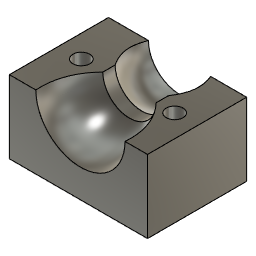
Arm0_1 (Autodesk Fusion 360 design; units mm, degrees)
Autodesk Fusion 360 part; units mm, degrees
note: some values were not read from the file. Set by a fixed rule: which sketch regions a step uses.
sketch "Sketch1" plane through (0, 0, 0) normal (0, 0, 1) x (1, 0, 0)
  line L0 (0.0319, -0.0588) -> (7.7319, -0.0588)
  line L1 (0.0319, 17.6912) -> (0.0319, -0.0588)
  line L2 (0.0319, 17.6912) -> (5.3319, 17.6912)
  line L3 (0.0319, 8.7412) -> (4.5319, 8.7412)
  line L4 (4.5319, 10.9412) -> (0.0319, 10.9412)
  spline S0 degree 5 poles (5.3319, 17.6912) (5.3878, 17.5532) (5.4935, 17.2775) (5.633, 16.8647) (5.7805, 16.3159) (5.8962, 15.6328) (5.9374, 14.9527) (5.8981, 14.2761) (5.7753, 13.6028) (5.5729, 12.9329) (5.297, 12.2661) (5.0223, 11.7348) (4.7879, 11.3376) (4.6193, 11.0732) (4.5319, 10.9412) knots 0 0 0 0 0 0 0.1 0.2 0.3 0.4 0.5 0.6 0.7 0.8 0.9 1 1 1 1 1 1
  line L5 (0.0319, 10.9412) -> (4.5319, 10.9412)
  arc A0 (7.7319, -0.0588) -> (4.5319, 8.7412) centre (-3.0926, 0.9869) ccw
  line L6 (4.5319, 8.7412) -> (4.5319, 10.9412)
  line L7 (0.0319, 10.9412) -> (0.0319, 8.7412)
  line L8 (0.0319, 10.9412) -> (0.0319, 8.7412)
  line L9 (0.0319, 14.3162) -> (5.8819, 14.3162)
  line L10 (0.0319, 17.6912) -> (0.0319, 10.9412)
  line L11 (7.7319, -0.0588) -> (7.9819, -0.0588)
  line L12 (4.5319, 8.7412) -> (4.7819, 8.7412)
  line L13 (4.5319, 10.9412) -> (4.7819, 10.9412)
  line L14 (5.8819, 14.3162) -> (6.1319, 14.3162)
  line L15 (5.3319, 17.6912) -> (5.5819, 17.6912)
  spline S1 degree 5 poles (5.5819, 17.6912) (5.6378, 17.5532) (5.7435, 17.2775) (5.883, 16.8647) (6.0305, 16.3159) (6.1462, 15.6328) (6.1874, 14.9527) (6.1481, 14.2761) (6.0253, 13.6028) (5.8229, 12.9329) (5.547, 12.2661) (5.2723, 11.7348) (5.0379, 11.3376) (4.8693, 11.0732) (4.7819, 10.9412) knots 0 0 0 0 0 0 0.1 0.2 0.3 0.4 0.5 0.6 0.7 0.8 0.9 1 1 1 1 1 1
  line L16 (4.7819, 10.9412) -> (4.7819, 8.7412)
  arc A1 (7.9819, -0.0588) -> (4.7819, 8.7412) centre (-2.9749, 0.9388) ccw
  line L17 (5.5819, 17.6912) -> (9, 17.6912)
  line L18 (9, 17.6912) -> (12, 17.6912)
  line L19 (12, 17.6912) -> (12, 0)
  line L20 (12, 0) -> (7.9819, -0.0588)
  dimension "d1" = 5.3
  dimension "d2" = 6.75
  dimension "d3" = 4.5
  dimension "d4" = 5.85
  dimension "d5" = 7.7
  dimension "d6" = 11
  dimension "d7" = 2.2
  dimension "d8" = 0.25
  dimension "d9" = 0.25
  dimension "d10" = 0.25
  dimension "d11" = 0.25
  dimension "d12" = 0.25
  constraint horizontal L2
  constraint perpendicular L2 L10
  constraint perpendicular L5 L10
  constraint midpoint L9.start L10
  constraint perpendicular L9 L10
  constraint horizontal L0
  constraint perpendicular L5 L8
  constraint horizontal L3
  constraint vertical L6
  constraint horizontal L4
  constraint vertical L7
  constraint perpendicular L0 L1
  constraint horizontal L11
  constraint horizontal L12
  constraint perpendicular L6 L13
  constraint horizontal L14
  constraint coincident L9.end L14.start
  constraint horizontal L15
  constraint tangent A0 A1
  constraint parallel L15 L17
  constraint parallel L17 L18
  constraint perpendicular L18 L19
  measures "d1" distance of L1.start L2.end
  measures "d2" distance of L4.end L1.start
  measures "d3" distance of L4.end L4.start
  measures "d4" distance of L9.end L9.start
  measures "d5" distance of L0.end L0.start
  measures "d6" distance of L4.end L0.start
  measures "d7" distance of L3.start L4.end
  measures "d8" distance of L0.end L11.end
  measures "d9" distance of L3.end L12.end
  measures "d10" distance of L4.start L13.end
  measures "d11" distance of L9.end L14.end
  measures "d12" distance of L2.end L15.end
revolve "Revolve1" add sketch "Sketch1" angle 360 about axis through (0.0319, 17.6912, 0) along (0, -1, 0) contours S1 L16 A1 L17 L18 L19 L20
sketch "Sketch2" plane through (0, 0, 0) normal (1, 0, 0) x (0, 1, 0)
  line L0 (25.8736, 15.4962) -> (-4, 15.4962)
  line L1 (-4, 15.4962) -> (-4, 0)
  line L2 (-4, 0) -> (25.8736, 0)
  line L3 (25.8736, 0) -> (25.8736, 15.4962)
  constraint horizontal L0
  constraint vertical L1
  constraint horizontal L2
  constraint vertical L3
extrude "Extrude1" cut sketch "Sketch2" along normal mid plane 100
sketch "Sketch3" plane through (0, 17.6912, 0) normal (0, 1, 0) x (-1, 0, 0)
  line L0 (11.9363, 0) -> (5.5181, 0)
  arc A0 (-5.5819, 0) -> (5.5181, 0) centre (-0.0319, 0) ccw
  line L1 (-5.5819, 0) -> (-12, 0)
  arc A1 (-12, 0) -> (11.9363, 0) centre (-0.0319, 0) ccw
  line L2 (-12, 0) -> (12.6512, 0)
  line L3 (12.6512, 0) -> (12.6512, -13)
  line L4 (12.6512, -13) -> (-12, -13)
  line L5 (-12, -13) -> (-12, 0)
  circle A2 centre (-0.0319, 0) radius 5.55
  dimension "d16" = 13
  constraint horizontal L2
  constraint vertical L3
  constraint horizontal L4
  constraint vertical L5
  constraint coincident L1.end A1.start
  constraint concentric A0 A2
  measures "d16" distance of L1.end L4.end
extrude "Extrude2" add sketch "Sketch3" against normal blind 17.691 contours A1 L2 L3 L4 L5
sketch "Sketch4" plane through (12, 0, 0) normal (1, 0, 0) x (0, 1, 0)
  line L0 (17.6912, -13) -> (17.6912, 0)
  line L1 (17.6912, 0) -> (0.0002, 0)
  line L2 (0.0002, 0) -> (0.0002, -13)
  line L3 (0.0002, -13) -> (17.6912, -13)
  line L4 (0.0002, 0) -> (-2.6841, 0)
  line L5 (-2.6841, 0) -> (-2.6841, -13)
  line L6 (-2.6841, -13) -> (0.0002, -13)
  line L7 (0.0002, -13) -> (0.0002, 0)
  constraint horizontal L4
  constraint vertical L5
  constraint horizontal L6
  constraint vertical L7
  constraint coincident L1.end L2.start
extrude "Extrude3" cut sketch "Sketch4" along normal mid plane 200 contours L2 L4 L5 L6 L7
sketch "Sketch5" plane through (0, 0, 0) normal (0, 0, 1) x (-1, 0, 0)
  line L0 (12.6512, -0.0002) -> (7.9234, -0.0002)
  arc A0 (4.7181, -8.7412) -> (7.9234, -0.0002) centre (-3.0386, -0.9388) ccw
  line L1 (4.7181, -8.7412) -> (4.7181, -10.9412)
  spline S0 degree 3 poles (5.5181, -17.6912) (5.7729, -17.0634) (5.9669, -16.3949) (6.1465, -14.9938) (6.1035, -14.3577) (5.7383, -12.6271) (5.1773, -11.6346) (4.7181, -10.9412) knots -0.494391 -0.494391 -0.494391 -0.494391 -0.376445 -0.376445 -0.249507 -0.249507 0 0 0 0
  line L2 (5.5181, -17.6912) -> (12.6512, -17.6912)
  line L3 (12.6512, -17.6912) -> (12.6512, -0.0002)
  line L4 (12.6512, -17.6912) -> (12.6512, -0.0002)
  line L5 (12.6512, -8.8457) -> (-12, -8.8457)
  line L6 (-12, -8.8457) -> (-12, -17.6912)
  circle A1 centre (8.6512, -8.8457) radius 1.5
  circle A2 centre (-8, -8.8457) radius 1.5
  dimension "d21" = 3
  dimension "d22" = 3
  dimension "d23" = 4
  dimension "d24" = 4
  constraint coincident L2.end L3.start
  constraint coincident L0.start L3.end
  constraint midpoint L4 L5.start
  constraint perpendicular L4 L5
  constraint perpendicular L5 L6
  constraint coincident L5 A1.centre
  constraint coincident L5 A2.centre
  measures "d21" diameter of A1
  measures "d22" diameter of A2
  measures "d23" distance of L5.end A2.centre
  measures "d24" distance of L5.start A1.centre
extrude "Extrude4" cut sketch "Sketch5" against normal through all contours L5 A1 | L5 A1 | L5 A2 | L5 A2
